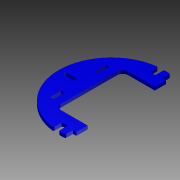
# Autodesk Inventor part: OpenROV 2.3 Dev EChassis Blinder
Saved by Autodesk Inventor 2012 (Build 160160000, 160)
## iProperties
Created: 2011-12-20
Part Number: OpenROV 2.3 Dev EChassis Blinder
Document SubType Name: Modeling
Designer: user
Density: 1 g/cm^3
Material: Default
Author: user
Autodesk Inventor part; units mm, degrees
ref_plane "YZ Plane" through (0, 0, 0) normal (1, 0, 0) x (0, 1, 0)
ref_plane "XZ Plane" through (0, 0, 0) normal (0, 1, 0) x (-1, 0, 0)
ref_plane "XY Plane" through (0, 0, 0) normal (0, 0, 1) x (1, 0, 0)
sketch "Sketch1" plane through (0, 0, 0) normal (0, 0, 1) x (1, 0, 0)
  line L0 (5.725, 40) -> (8.725, 40)
  line L1 (8.725, 40) -> (8.725, 30)
  line L2 (8.725, 30) -> (-15, 30)
  line L3 (5.725, -40) -> (8.725, -40)
  line L4 (8.725, -40) -> (8.725, -30)
  line L5 (8.725, -30) -> (-15, -30)
  line L6 (5.725, 45.7567) -> (5.725, 40)
  line L7 (-20, 25) -> (-20, -25)
  line L8 (5.725, -40) -> (5.725, -45.7567)
  arc A0 (5.725, 45.7567) -> (4.8277, 46.7514) centre (4.725, 45.7567) ccw
  arc A1 (4.8277, -46.7514) -> (5.725, -45.7567) centre (4.725, -45.7567) ccw
  line L9 (-30, 25) -> (-27, 25)
  line L10 (-27, 25) -> (-27, 15)
  line L11 (-27, 15) -> (-30, 15)
  line L12 (-30, 15) -> (-30, 25)
  line L13 (-30, -15) -> (-27, -15)
  line L14 (-27, -15) -> (-27, -25)
  line L15 (-27, -25) -> (-30, -25)
  line L16 (-30, -25) -> (-30, -15)
  arc A2 (-15, 30) -> (-20, 25) centre (-15, 25) ccw
  arc A3 (-20, -25) -> (-15, -30) centre (-15, -25) ccw
  line L17 (-42, 1.5) -> (-32, 1.5)
  line L18 (-32, 1.5) -> (-32, -1.5)
  line L19 (-32, -1.5) -> (-42, -1.5)
  line L20 (-42, -1.5) -> (-42, 1.5)
  line L21 (0, -45.9891) -> (0, -40)
  line L22 (-1, -39) -> (-4, -39)
  line L23 (-5, -40) -> (-5, -45.607)
  arc A4 (1.0217, -46.9889) -> (4.8277, -46.7514) centre (0, 0) ccw
  line L24 (0, 45.9891) -> (0, 40)
  line L25 (-1, 39) -> (-4, 39)
  line L26 (-5, 40) -> (-5, 45.607)
  arc A5 (4.8277, 46.7514) -> (1.0217, 46.9889) centre (0, 0) ccw
  arc A6 (-6.1304, 46.5985) -> (-6.1304, -46.5985) centre (0, 0) ccw
  arc A7 (-5, 45.607) -> (-6.1304, 46.5985) centre (-6, 45.607) ccw
  arc A8 (1.0217, 46.9889) -> (0, 45.9891) centre (1, 45.9891) ccw
  arc A9 (-1, 39) -> (0, 40) centre (-1, 40) ccw
  arc A10 (-5, 40) -> (-4, 39) centre (-4, 40) ccw
  arc A11 (-6.1304, -46.5985) -> (-5, -45.607) centre (-6, -45.607) ccw
  arc A12 (-4, -39) -> (-5, -40) centre (-4, -40) ccw
  arc A13 (0, -40) -> (-1, -39) centre (-1, -40) ccw
  arc A14 (0, -45.9891) -> (1.0217, -46.9889) centre (1, -45.9891) ccw
  point P0 (5.725, 46.65)
  point P1 (5.725, -46.65)
  point P2 (0, -47)
  point P3 (0, -39)
  point P4 (-5, -39)
  point P5 (-5, -46.7333)
  point P6 (0, 47)
  point P7 (0, 39)
  point P8 (-5, 39)
  point P9 (-5, 46.7333)
  dimension "d2" = 10
  dimension "d3" = 30
  dimension "d4" = 30
  dimension "d5" = 10
  dimension "d8" = 1
  dimension "d9" = 3
  dimension "d10" = 3
  dimension "d12" = 10
  dimension "d13" = 15
  dimension "d14" = 15
  dimension "d15" = 30
  dimension "d16" = 30
  dimension "d18" = 3
  dimension "d19" = 3
  dimension "d20" = 20
  dimension "d21" = 5
  dimension "d26" = 3
  dimension "d27" = 10
  dimension "d29" = 1.5
  dimension "d48" = 10
  dimension "d51" = 32
  dimension "d52" = 8
  dimension "d53" = 5
  dimension "d54" = 7.7333
  dimension "d55" = 8
  dimension "d56" = 5
  dimension "d57" = 7.7333
  dimension "d58" = 1
  constraints: 54 end point, 34 point on circle, 22 tangent, 15 centre point, 14 point on line, 11 parallel, 9 equal radius, 8 perpendicular, 5 horizontal, 3 vertical, 1 coincident
  measures "d2" distance of L0.end L1.end
  measures "d3" distance from line of point (0, 0) L2
  measures "d4" distance from line of point (0, 0) L5
  measures "d5" distance of L3.end L4.end
  measures "d8" radius of A0
  measures "d9" distance of L10.end L11.end
  measures "d10" distance of L13.start L13.end
  measures "d12" distance of L11.end L9.start
  measures "d13" distance from line of point (0, 0) L11
  measures "d14" distance from line of point (0, 0) L13
  measures "d15" distance from line of point (0, 0) L12
  measures "d16" distance from line of point (0, 0) L16
  measures "d18" distance of L0.start L0.end
  measures "d19" distance of L3.start L3.end
  measures "d20" distance from line of point (0, 0) L7
  measures "d21" radius of A2
  measures "d26" distance of L19.end L17.start
  measures "d27" distance of L17.start L17.end
  measures "d29" distance from line of point (0, 0) L17
  measures "d48" distance of L15.end L13.start
  measures "d51" distance from line of point (0, 0) L18
  measures "d52" distance of point (0, -47) point (0, -39)
  measures "d53" distance of point (0, -39) point (-5, -39)
  measures "d54" distance of point (-5, -39) point (-5, -46.733)
  measures "d55" distance of point (0, 47) point (0, 39)
  measures "d56" distance of point (0, 39) point (-5, 39)
  measures "d57" distance of point (-5, 39) point (-5, 46.733)
  measures "d58" radius of A7
extrude "Extrusion2" add sketch "Sketch1" along normal blind 3
body "Solid2"
